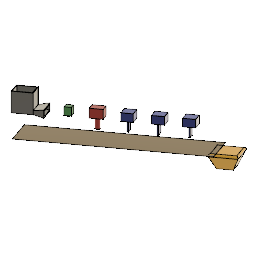
ChopperSubsystemRoughOutline Version2 (Autodesk Fusion 360 design; units mm, degrees)
Autodesk Fusion 360 part; units mm, degrees
sketch "ConveryorBelt" plane through (0, 0, 0) normal (0, 0, 1) x (1, 0, 0)
  line L0 (-1500, 1000) -> (7550, 1000)
  line L1 (7550, 1000) -> (7550, -1000)
  line L2 (7550, -1000) -> (-1500, -1000)
  line L3 (-1500, -1000) -> (-1500, 1000)
  dimension "d1" = 9050
  dimension "d2" = 2000
  constraint horizontal L0
  constraint vertical L1
  constraint horizontal L2
  constraint vertical L3
  measures "d1" distance of L0.start L0.end
  measures "d2" distance of L0.end L1.end
sketch "VegetableStorage/Dropping" plane through (0, 0, 0) normal (0, 0, 1) x (1, 0, 0)
  line L0 (-1700, 416.3983) -> (-702.4107, 416.3983)
  line L1 (-702.4107, 416.3983) -> (-702.4107, -450)
  line L2 (-702.4107, -450) -> (-1700, -450)
  line L3 (-1700, -450) -> (-1700, 416.3983)
  constraint horizontal L0
  constraint vertical L1
  constraint horizontal L2
  constraint vertical L3
extrude "Extrude1" add sketch "ConveryorBelt" along normal blind 3 makes body 1
extrude "Extrude2" add sketch "VegetableStorage/Dropping" along normal blind 1000 from surface at 1000 separate body makes body 2
shell "Shell1" thickness 40 removed faces 1 at (-1367.4702, 127.5989, 2000) on bodies 2
sketch "VegetableStorageProtrusion" plane through (-702.4107, 0, 0) normal (1, 0, 0) x (0, 1, 0)
  line L0 (-450, 1000) -> (416.3983, 1000)
  line L1 (416.3983, 1000) -> (416.3983, 2000)
  line L2 (416.3983, 2000) -> (-450, 2000)
  line L3 (-450, 2000) -> (-450, 1000)
  line L4 (-450, 1200) -> (416.3983, 1200)
  line L5 (416.3983, 1200) -> (416.3983, 1000)
  line L6 (416.3983, 1000) -> (-450, 1000)
  line L7 (-450, 1000) -> (-450, 1200)
  constraint horizontal L4
  constraint vertical L5
  constraint horizontal L6
  constraint vertical L7
  constraint collinear L1 L5
  constraint collinear L3 L7
  constraint collinear L0 L6
extrude "Extrude3" add sketch "VegetableStorageProtrusion" along normal blind 500 draft 10 contours L0 L1 L3 L4 L5 L6 L7 bodies 2
shell "Shell2" thickness 60 removed faces 1 at (-202.4107, 156.9867, 1037.2788) on bodies 2
sketch "ComputerVisionCamera" plane through (0, 0, 3) normal (0, 0, 1) x (-1, 0, 0)
  line L0 (1500, 1000) -> (-7550, 1000)
  line L1 (-7550, 1000) -> (-7550, -1000)
  line L2 (-7550, -1000) -> (1500, -1000)
  line L3 (1500, -1000) -> (1500, 1000)
  line L4 (-600, -172.6758) -> (-947.5188, -172.6758)
  line L5 (-947.5188, -172.6758) -> (-947.5188, 174.843)
  line L6 (-947.5188, 174.843) -> (-600, 174.843)
  line L7 (-600, 174.843) -> (-600, -172.6758)
  constraint horizontal L4
  constraint vertical L5
  constraint horizontal L6
  constraint vertical L7
  constraint equal L5 L6
extrude "Extrude5" add sketch "ComputerVisionCamera" along normal blind 400 from surface at 1000 separate body contours L4 L5 L6 L7 makes body 3
sketch "CameraExtension" plane through (0, 0, 1003) normal (0, 0, -1) x (1, 0, 0)
  line L0 (947.5188, 174.843) -> (600, 174.843)
  line L1 (600, 174.843) -> (600, -172.6758)
  line L2 (600, -172.6758) -> (947.5188, -172.6758)
  line L3 (947.5188, -172.6758) -> (947.5188, 174.843)
  circle A0 centre (773.7594, 1.0836) radius 77.5643
  line L4 (773.7594, 174.843) -> (773.7594, -172.6758)
  point P0 (773.7594, 1.0836)
  constraint midpoint L0 L4.start
  constraint midpoint L2 L4.end
  constraint midpoint L4 P0
  constraint coincident P0 A0.centre
extrude "Extrude6" add sketch "CameraExtension" along normal blind 60 contours A0 L4 | A0 L4 bodies 3
sketch "PrepMachine" plane through (0, 0, 3) normal (0, 0, 1) x (-1, 0, 0)
  line L0 (1500, 1000) -> (-7550, 1000)
  line L1 (-7550, 1000) -> (-7550, -1000)
  line L2 (-7550, -1000) -> (1500, -1000)
  line L3 (1500, -1000) -> (1500, 1000)
  line L4 (202.4107, -443.6362) -> (202.4107, 477.2379)
  line L5 (-1749.5188, -250) -> (-2387.8803, -250)
  line L6 (-2387.8803, -250) -> (-2387.8803, 250)
  line L7 (-2387.8803, 250) -> (-1749.5188, 250)
  line L8 (-1749.5188, 250) -> (-1749.5188, -250)
  line L9 (-947.5188, -172.6758) -> (-947.5188, 174.843)
  point P0 (-600, -172.6758)
  constraint horizontal L5
  constraint vertical L6
  constraint horizontal L7
  constraint vertical L8
extrude "Extrude8" add sketch "PrepMachine" along normal blind 460 from surface at 1000 separate body contours L5 L6 L7 L8 makes body 4
sketch "PrepMachine-Decore" plane through (0, 0, 1003) normal (0, 0, -1) x (1, 0, 0)
  line L0 (2387.8803, 250) -> (1749.5188, 250)
  line L1 (1749.5188, 250) -> (1749.5188, -250)
  line L2 (1749.5188, -250) -> (2387.8803, -250)
  line L3 (2387.8803, -250) -> (2387.8803, 250)
  circle A0 centre (2068.6995, -1.0765) radius 122.2133
  circle A1 centre (2068.6995, -1.0765) radius 80.1333
  constraint concentric A0 A1
extrude "Extrude9" add sketch "PrepMachine-Decore" along normal blind 520 contours A0 bodies 4
fillet "Fillet1" radius 15 1 edges at (701.4441, 26.9648, 943) on bodies 3
sketch "Chopper" plane through (0, 0, 3) normal (0, 0, 1) x (-1, 0, 0)
  line L0 (-3189.8803, -300) -> (-3757.1142, -300)
  line L1 (-3757.1142, -300) -> (-3757.1142, 300)
  line L2 (-3757.1142, 300) -> (-3189.8803, 300)
  line L3 (-3189.8803, 300) -> (-3189.8803, -300)
  line L4 (-2387.8803, -250) -> (-2387.8803, 250)
  line L5 (-3189.8803, -300) -> (-3757.1142, -300)
  line L6 (-3757.1142, 300) -> (-3189.8803, 300)
  line L7 (-3757.1142, -300) -> (-3757.1142, 300)
  line L8 (-4559.1142, -300) -> (-5159.1142, -300)
  line L9 (-5159.1142, -300) -> (-5159.1142, 300)
  line L10 (-5159.1142, 300) -> (-4559.1142, 300)
  line L11 (-4559.1142, 300) -> (-4559.1142, -300)
  line L12 (-5961.1142, -300) -> (-6561.1142, -300)
  line L13 (-6561.1142, -300) -> (-6561.1142, 300)
  line L14 (-6561.1142, 300) -> (-5961.1142, 300)
  line L15 (-5961.1142, 300) -> (-5961.1142, -300)
  constraint horizontal L0
  constraint vertical L1
  constraint horizontal L2
  constraint vertical L3
  constraint horizontal L5
  constraint vertical L7
  constraint horizontal L6
  constraint horizontal L8
  constraint vertical L9
  constraint horizontal L10
  constraint vertical L11
  constraint horizontal L12
  constraint vertical L13
  constraint horizontal L14
  constraint vertical L15
extrude "Extrude10" add sketch "Chopper" along normal blind 400 from surface at 1000 separate body makes body 5 at (3378.9583, 100, 1003) makes body 6 at (4959.1142, 100, 1003) makes body 7 at (6161.1142, 100, 1003)
sketch "ChopperBlades" plane through (0, 0, 1003) normal (0, 0, -1) x (1, 0, 0)
  line L0 (3757.1142, 300) -> (3189.8803, 300)
  line L1 (3189.8803, 300) -> (3189.8803, -300)
  line L2 (3189.8803, -300) -> (3757.1142, -300)
  line L3 (3757.1142, -300) -> (3757.1142, 300)
  line L4 (3509.8055, 179.6391) -> (3439.8055, 179.6391)
  line L5 (3439.8055, 179.6391) -> (3439.8055, -140)
  line L6 (3439.8055, -140) -> (3510.6881, -140)
  line L7 (3510.6881, -140) -> (3509.8055, 179.6391)
  line L8 (3513.9634, -140.0014) -> (3513.9634, 259.9986)
  line L9 (4808.3191, -140) -> (4879.2016, -140)
  line L10 (4879.2016, -140) -> (4879.2016, 260)
  line L11 (4879.2016, 260) -> (4808.3191, 260)
  line L12 (4808.3191, 260) -> (4808.3191, -140)
  line L13 (6212.8571, -140) -> (6282.8571, -140)
  line L14 (6282.8571, -140) -> (6282.8571, 179.6403)
  line L15 (6282.8571, 179.6403) -> (6212.8571, 179.6403)
  line L16 (6212.8571, 179.6403) -> (6212.8571, -140)
  line L17 (5159.1142, -300) -> (4559.1142, -300)
  line L18 (6561.1142, -300) -> (5961.1142, -300)
  constraint horizontal L4
  constraint vertical L5
  constraint horizontal L6
  constraint horizontal L9
  constraint vertical L10
  constraint horizontal L11
  constraint vertical L12
  constraint horizontal L13
  constraint vertical L14
  constraint horizontal L15
  constraint vertical L16
  constraint equal L6 L9
  constraint equal L4 L15
  constraint equal L8 L10
  constraint equal L7 L14
extrude "Extrude11" add sketch "ChopperBlades" along normal blind 500 contours L4 L5 L6 L7 | L9 L10 L11 L12 | L13 L14 L15 L16 bodies 5 6 7
sketch "ChoppedVeggieCollector" plane through (0, 0, 0) normal (0, 0, 1) x (1, 0, 0)
  line L0 (7157.3316, 731.5275) -> (8620.3869, 731.5275)
  line L1 (8620.3869, 731.5275) -> (8620.3869, -731.5277)
  line L2 (8620.3869, -731.5277) -> (7157.3316, -731.5277)
  line L3 (7157.3316, -731.5277) -> (7157.3316, 731.5275)
  line L4 (3757.1142, 300) -> (3757.1142, -300)
  line L5 (7157.3316, 731.5275) -> (8620.3869, -731.5277)
  line L6 (8620.3869, 731.5275) -> (7157.3316, -731.5277)
  line L7 (1.75, 0) -> (22.5, 0)
  line L8 (6355.3316, 325.5378) -> (6355.3316, 526.2213)
  point P0 (7888.8593, -0.0001)
  constraint horizontal L0
  constraint vertical L1
  constraint horizontal L2
  constraint vertical L3
  constraint perpendicular L5 L6
  constraint midpoint L5 P0
  constraint parallel L1 L8
extrude "Extrude12" add sketch "ChoppedVeggieCollector" along normal blind 0 draft 20 and the other way blind 750 draft -25 separate body makes body 8
fillet "Fillet2" radius 90 1 faces at (7645.0167, -243.8426, 0) on bodies 8
equation "d1 = 8.15 m + 0.9 m"
named bodies: "ConveyorBElt", "VegetableStorer/Dropper", "ComputerVisionCamera", "Prep&Decore", "Chopper", "ChoppedVeggieCollector"
